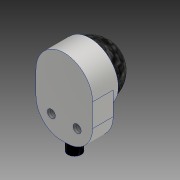
# Autodesk Inventor part: OptoForce_OMD-10-SE-10N
Saved by Autodesk Inventor 2017 SP1 (Build 210196100, 196)
## iProperties
Created: 2017-06-27
Part Number: OptoForce_OMD-10-SE-10N
Material: Generic
Document SubType Name: Modeling
Designer: Tomasz
Density: 1 g/cm^3
Appearance: Aluminum - Flat
Author: Tomasz
Autodesk Inventor part; units mm, degrees
ref_plane "YZ Plane" through (0, 0, 0) normal (1, 0, 0) x (0, 1, 0)
sketch "Sketch1" plane through (0, 0, 0) normal (0, 1, 0) x (-1, 0, 0)
  arc A0 (5.5, 0) -> (-5.5, 0) centre (0, 0) ccw
  line L0 (5.5, 0) -> (5.5, -4.5)
  line L1 (-5.5, 0) -> (-5.5, -4.5)
  line L2 (-0.5, -9.5) -> (0.5, -9.5)
  arc A1 (-5.5, -4.5) -> (-0.5, -9.5) centre (-0.5, -4.5) ccw
  arc A2 (0.5, -9.5) -> (5.5, -4.5) centre (0.5, -4.5) ccw
  line L3 (0, 0) -> (0, -9.5) construction
  dimension "d0" = 11
  dimension "d1" = 15
  dimension "d2" = 5
  constraints: 8 end point, 6 point on circle, 6 tangent, 3 centre point, 2 vertical, 1 coincident, 1 equal radius, 1 midpoint, 1 perpendicular
  measures "d0" diameter of A0
  measures "d2" radius of A1
extrude "Extrusion1" add sketch "Sketch1" along normal blind 4
sketch "Sketch2" plane through (0, 4, 0) normal (0, 1, 0) x (1, 0, 0)
  circle A0 centre (0, 0) radius 5.5
  arc A1 (-5.5, 0) -> (5.5, 0) centre (0, 0) ccw projected
  constraints: 1 centre point, 1 coincident, 1 concentric
extrude "Extrusion2" add sketch "Sketch2" along normal blind 1
ref_plane "Work Plane1" through (0, 0, 0) normal (1, 0, 0) x (0, 0, -1)
sketch "Sketch4" plane through (0, 0, 0) normal (1, 0, 0) x (0, 0, -1)
  line L0 (5.5, 5) -> (-5.5, 5) projected
  line L1 (0, 5) -> (0, 11.0328) construction
  arc A0 (5, 5) -> (0, 10) centre (0, 5) ccw
  line L2 (0, 10) -> (0, 5)
  line L3 (0, 5) -> (5, 5)
  point P0 (0, 0)
  dimension "d8" = 5
  constraints: 6 end point, 2 point on circle, 2 vertical, 1 centre point, 1 coincident, 1 midpoint, 1 perpendicular, 1 point on line
  measures "d8" distance of L2.start L1.start
revolve "Revolution1" add sketch "Sketch4" angle 360 about axis through (0, 5, 0) along (0, 1, 0)
sketch "Sketch5" plane through (0, 0, 0) normal (0, -1, 0) x (1, 0, 0)
  line L0 (0, 0) -> (0, -9.4931) construction
  point P0 (2.5, -6)
  point P1 (-2.5, -6)
  dimension "d10" = 6
  dimension "d11" = 5
  constraints: 2 end point, 1 symmetric about line, 1 vertical
  measures "d10" vertical distance of point (2.5, -6) L0.start
  measures "d11" distance of point (-2.5, -6) point (2.5, -6)
hole "Hole1" at (2.5, 0, -6) at (-2.5, 0, -6) direction (0, 1, 0) diameter 1.567 end through all thread size "M2x0.4" class "6H" standard "ANSI Metric M Profile"
ref_plane "Work Plane2" through (0.5, 0, -9) normal (0, 0, -1) x (-1, 0, 0)
sketch "Sketch6" plane through (0.5, 0, -9) normal (0, 0, -1) x (-1, 0, 0)
  line L0 (0, 0) -> (1, 0) projected
  line L1 (1, 0) -> (1, 4) projected
  line L2 (0, 4) -> (1, 4) projected
  line L3 (0, 0) -> (0, 4) projected
  line L4 (0, 0) -> (0, 4) projected
  line L5 (0, 2) -> (1, 2) construction
  line L6 (1, 0) -> (1, 4) projected
  circle A0 centre (0.5, 2) radius 1.3
  point P0 (0.5, 0)
  dimension "d20" = 2.6
  constraints: 3 midpoint, 2 end point, 1 centre point
  measures "d20" diameter of A0
extrude "Extrusion3" add sketch "Sketch6" along normal blind 3 contours A0 L3 | L3 A0 L1 | L1 A0
body "Solid1"
